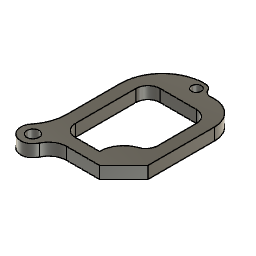
draw 1 v1 (Autodesk Fusion 360 design; units mm, degrees)
Autodesk Fusion 360 part; units mm, degrees
sketch "Sketch1" plane through (0, 0, 0) normal (0, 0, 1) x (1, 0, 0)
  circle A0 centre (-0.0001, 0.0013) radius 1
  line L0 (14, 16) -> (14, 5)
  line L1 (4, 17) -> (10, 17)
  line L2 (12, 15) -> (12, 8.6569)
  line L3 (8, 3) -> (4, 3)
  line L4 (2, 5) -> (2, 15)
  circle A1 centre (6.9999, 20) radius 0.8
  line L5 (10, 1) -> (14, 5)
  line L6 (12, 1) -> (15.2632, 1) construction
  arc A2 (10.6667, 6.7712) -> (8, 3) centre (12, 3) ccw
  arc A3 (4, 17) -> (2, 15) centre (4, 15) ccw
  arc A4 (12, 15) -> (10, 17) centre (10, 15) ccw
  arc A5 (2, 5) -> (4, 3) centre (4, 5) ccw
  arc A6 (10.6667, 6.7712) -> (12, 8.6569) centre (10, 8.6569) ccw
  line L7 (14, 15) -> (14, 8.6569)
  line L8 (10, 1) -> (4, 1)
  line L9 (0, 5) -> (0, 15)
  arc A7 (-1.5556, 1.2584) -> (1.8327, -0.7992) centre (-0.0001, 0.0013) ccw
  line L10 (0, 1) -> (0, 1.0013)
  line L11 (0, 5.6582) -> (0, 14.4)
  line L12 (10, 1) -> (4.582, 1)
  line L13 (0.0503, 1) -> (0, 1)
  arc A8 (-1.5556, 1.2584) -> (0, 5.6582) centre (-7, 5.6582) ccw
  arc A9 (4.582, 1) -> (1.8327, -0.7992) centre (4.582, -2) ccw
  arc A10 (6.9999, 21.4) -> (0, 14.4) centre (7, 14.4) ccw
  arc A11 (7, 21.4) -> (6.9999, 21.4) centre (6.9999, 20) ccw
  line L14 (10, 20) -> (9.1816, 20)
  arc A12 (8.2726, 20.5833) -> (6.9999, 21.4) centre (6.9999, 20) ccw
  arc A13 (8.2726, 20.5833) -> (9.1816, 20) centre (9.1816, 21) ccw
  arc A14 (14, 16) -> (10, 20) centre (10, 16) ccw
  dimension "d1" = 4
  dimension "d2" = 2
  dimension "d3" = 1.6
  dimension "d4" = 2.8
  dimension "d5" = 14
  dimension "d8" = 20
  dimension "d10" = 17
  dimension "d11" = 15
  dimension "d12" = 3
  dimension "d13" = 8
  dimension "d14" = 2
  dimension "d15" = 2
  dimension "d16" = 2
  dimension "d17" = 2
  dimension "d19" = 7
  dimension "d20" = 3
  dimension "d21" = 7
  dimension "d23" = 1
  dimension "d24" = 4
  constraint concentric A0 A7
  constraint vertical L0
  constraint vertical L10
  constraint horizontal L1
  constraint vertical L2
  constraint horizontal L3
  constraint vertical L4
  constraint concentric A1 A11
  constraint horizontal L6
  constraint coincident origin L10
  constraint midpoint L5 A2.centre
  constraint tangent L1 A3
  constraint tangent L4 A3
  constraint tangent L1 A4
  constraint tangent L2 A4
  constraint tangent L3 A5
  constraint tangent L4 A5
  constraint equal A4 A5
  constraint tangent A2 A6
  constraint tangent L2 A6
  constraint equal A4 A6
  constraint parallel L2 L7
  constraint parallel L3 L8
  constraint parallel L4 L9
  constraint coincident A0 L10.end
  constraint collinear L10 L11
  constraint coincident A0 L13.start
  constraint collinear L12 L13
  constraint tangent L11 A8
  constraint tangent A7 A8
  constraint tangent L12 A9
  constraint tangent A7 A9
  constraint tangent L11 A10
  constraint tangent A10 A11
  constraint perpendicular L0 L14
  constraint concentric A1 A12
  constraint tangent A12 A13
  constraint tangent L14 A13
  constraint coincident A1.centre L14
  constraint tangent L14 A14
  constraint tangent L0 A14
  measures "d1" diameter of A7
  measures "d2" diameter of A0
  measures "d3" diameter of A1
  measures "d4" diameter of A11
  measures "d5" distance of origin L0
  measures "d8" vertical distance of origin A1.centre
  measures "d10" distance of L3 A1.centre
  measures "d11" vertical distance of A1.centre L0.end
  measures "d12" distance of L1 A1.centre
  measures "d13" diameter of A2
  measures "d14" distance of L4 L10
  measures "d15" distance of L0 L2
  measures "d16" radius of A3
  measures "d17" radius of A4
  measures "d19" radius of A8
  measures "d20" radius of A9
  measures "d21" radius of A10
  measures "d23" radius of A13
  measures "d24" radius of A14
extrude "Extrude1" add sketch "Sketch1" along normal blind 2
